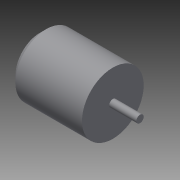
# Autodesk Inventor part: 5045motor
Saved by Autodesk Inventor 2014 (Build 180170000, 170)
## iProperties
Created: 2014-05-15
Part Number: 5045motor
Material: Generic
Document SubType Name: Modeling
Designer: brent
Density: 1 g/cm^3
Appearance: Default
d0: 0.984 in
d1: 2.323 in
d2: 0.118 in
d3: 0.866 in
d5: 0.200 in
Author: brent
Autodesk Inventor part; units mm, degrees
ref_plane "YZ Plane" through (0, 0, 0) normal (1, 0, 0) x (0, 1, 0)
ref_plane "XZ Plane" through (0, 0, 0) normal (0, 1, 0) x (-1, 0, 0)
ref_plane "XY Plane" through (0, 0, 0) normal (0, 0, 1) x (1, 0, 0)
sketch "Sketch1" plane through (0, 0, 0) normal (0, 0, 1) x (1, 0, 0)
  line L0 (-39.7038, 0) -> (73.6962, 0) projected
  line L1 (-23.5038, 0) -> (35.4962, 0)
  line L2 (35.4962, 0) -> (35.4962, 25)
  line L3 (35.4962, 25) -> (-23.5038, 25)
  line L4 (-23.5038, 25) -> (-23.5038, 0)
  line L5 (35.4962, 3) -> (57.4962, 3)
  line L6 (57.4962, 3) -> (57.4962, 0)
  line L7 (57.4962, 0) -> (35.4962, 0)
  line L8 (35.4962, 0) -> (35.4962, 3)
  point P0 (0, 0)
  dimension "d0" = 25
  dimension "d1" = 59
  dimension "d2" = 3
  dimension "d3" = 22
  constraints: 16 end point, 4 parallel, 3 point on line, 2 horizontal, 2 perpendicular
  measures "d0" distance between parallel lines of L1 L3
  measures "d1" distance between parallel lines of L2 L4
  measures "d2" distance between parallel lines of L7 L5
  measures "d3" distance between parallel lines of L2 L6
revolve "Revolution1" add sketch "Sketch1" angle 360 about axis through (-23.5038, 0, 0) along (1, 0, 0)
chamfer "Chamfer1" distance 5.08 angle 45 1 edges at (-23.5038, -25, 0)
body "Solid1"
